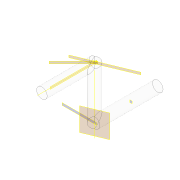
# Autodesk Inventor part: 00_Beam_Ocular_Detectoin
Saved by Autodesk Inventor 2019 (Build 230136000, 136)
## iProperties
Created: 2019-11-14
Part Number: 00_Beam_Ocular_Detectoin
Material: Generic
Document SubType Name: Modeling
Designer: diederichbenedict
Density: 1 g/cm^3
Appearance: Polycarbonate - Clear
Author: diederichbenedict
Autodesk Inventor part; units mm, degrees
ref_plane "XZ Plane" through (0, 0, 0) normal (0, 1, 0) x (-1, 0, 0)
ref_plane "XY Plane" through (0, 0, 0) normal (0, 0, 1) x (1, 0, 0)
sketch "Sketch1" plane through (0, 0, 0) normal (0, 0, 1) x (1, 0, 0)
  circle A0 centre (0, 0) radius 5
  dimension "d0" = 10
  constraints: 1 centre point, 1 coincident
  measures "d0" diameter of A0
extrude "Extrusion1" add sketch "Sketch1" against normal blind 50
ref_plane "Work Plane1" through (0, 0, -50) normal (0, 0, -1) x (-1, 0, 0)
ref_plane "Work Plane3" through (0, 0, -50) normal (0.7071068, 0, 0.7071068) x (0, -1, 0)
ref_plane "Work Plane2" through (0, 0, -50) normal (1, 0, 0) x (0, 1, 0)
sketch "Sketch2" plane through (0, 0, -50) normal (0.7071068, 0, 0.7071068) x (0, -1, 0)
  ellipse E0 centre (0, 0) end of major axis (-5, 0) minor radius 3.5355 projected
  circle A0 centre (0, 0) radius 5
  point P0 (0, -35.3553)
  dimension "d14" = 10
  constraints: 1 centre point, 1 coincident, 1 other
  measures "d14" diameter of A0
extrude "Extrusion2" add sketch "Sketch2" along normal blind 70
ref_plane "Work Plane4" through (49.4975, 0, -0.5025) normal (0, 0, -1) x (-1, 0, 0)
sketch "Sketch3" plane through (49.4975, 0, -0.5025) normal (0, 0, -1) x (-1, 0, 0)
  ellipse E0 centre (0, 0) end of major axis (0, 5) minor radius 3.5355 projected
  circle A0 centre (0, 0) radius 5
  point P0 (49.4975, 0)
  constraints: 1 centre point, 1 coincident, 2 other
extrude "Extrusion3" add sketch "Sketch3" along normal blind 60
ref_plane "Work Plane5" through (0, 0, -50) normal (0.3826834, 0, 0.9238795) x (0, -1, 0)
sketch "Sketch4" plane through (0, 0, -50) normal (0.3826834, 0, 0.9238795) x (0, -1, 0)
  circle A0 centre (0, 0) radius 2.8545
  point P0 (0, -19.1342)
  constraints: 1 centre point
extrude "Extrusion4" add sketch "Sketch4" along normal blind 1
ref_plane "Work Plane8" through (49.4975, 0, -0.5025) normal (0.3826834, 0, 0.9238795) x (0, 1, 0)
sketch "Sketch5" plane through (49.4975, 0, -0.5025) normal (0.3826834, 0, 0.9238795) x (0, 1, 0)
  circle A0 centre (0, 0) radius 2.6859
  point P0 (0, 45.922)
  constraints: 1 centre point, 1 coincident
extrude "Extrusion5" add sketch "Sketch5" against normal blind 1
ref_plane "Work Plane7" through (49.4975, 0, -35.0025) normal (0, 0, -1) x (-1, 0, 0)
sketch "Sketch6" plane through (49.4975, 0, -35.0025) normal (0, 0, -1) x (-1, 0, 0)
  ellipse E0 centre (0, 0) end of major axis (0, -2.6859) minor radius 2.4814 projected
  line L0 (-2.1727, -1.2973) -> (2.1727, -1.2973)
  line L1 (2.1727, -1.2973) -> (2.1727, 1.2973)
  line L2 (2.1727, 1.2973) -> (-2.1727, 1.2973)
  line L3 (-2.1727, 1.2973) -> (-2.1727, -1.2973)
  line L4 (0, -5) -> (0, 5) projected
  line L5 (-2.1727, -1.2973) -> (2.1727, 1.2973) construction
  line L6 (2.1727, -1.2973) -> (-2.1727, 1.2973) construction
  point P0 (49.4975, 0)
  point P1 (0, 0)
  constraints: 12 end point, 3 midpoint, 2 parallel, 1 horizontal, 1 perpendicular, 2 other
extrude "Extrusion6" add sketch "Sketch6" along normal blind 1 contours L0 L4 L2 L1 | L3 L2 L4 L0
body "Solid1"
